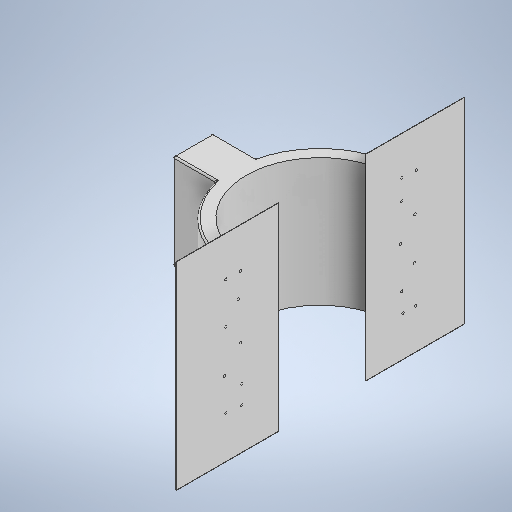
# Autodesk Inventor part: moror-mount1
Saved by Autodesk Inventor 2025.2 (Build 292293000, 293)
## iProperties
Created: 2025-02-07
Part Number: moror-mount1
Material: 一般
Document SubType Name: Modeling
Designer: mahhy
Density: 1 g/cm^3
Appearance: 既定
Author: mahhy
## iProperties of the stored document moror-mount1_3D プリント.ipt
Created: 2025-02-16
Part Number: moror-mount1_3D プリント
Material: 一般
Document SubType Name: Modeling
Designer: mahhy
Density: 1 g/cm^3
Appearance: 既定
Author: mahhy
Autodesk Inventor part; units mm, degrees
ref_plane "YZ Plane" through (0, 0, 0) normal (1, 0, 0) x (0, 1, 0)
ref_plane "XZ Plane" through (0, 0, 0) normal (0, 1, 0) x (-1, 0, 0)
ref_plane "XY Plane" through (0, 0, 0) normal (0, 0, 1) x (1, 0, 0)
sketch "スケッチ1" plane through (0, 0, 0) normal (0, 1, 0) x (-1, 0, 0)
  line L0 (0, 0) -> (60, 0)
  line L1 (60, 0) -> (60, -120)
  line L2 (60, -120) -> (0, -120)
  line L3 (0, -120) -> (0, 0)
  circle A0 centre (0, -60) radius 46
  circle A1 centre (0, -60) radius 54
  line L4 (0, -14) -> (7, -14)
  line L5 (7, -14) -> (7, 4)
  line L6 (7, 4) -> (0, 4)
  line L7 (0, 4) -> (0, -14)
  line L8 (0, -106) -> (7, -106)
  line L9 (7, -106) -> (7, -124)
  line L10 (7, -124) -> (0, -124)
  line L11 (0, -124) -> (0, -106)
  line L12 (54, -47.5) -> (46, -47.5)
  line L13 (46, -47.5) -> (46, -72.5)
  line L14 (46, -72.5) -> (54, -72.5)
  line L15 (54, -72.5) -> (54, -47.5)
  point P0 (46, -60)
  point P1 (52.5333, -47.5)
  point P2 (7, -6.4556)
  point P3 (0, -2)
  point P4 (0, -118)
  point P5 (7, -113.5444)
  point P6 (52.5333, -72.5)
  point P7 (7, 0)
  point P8 (7, -120)
  point P9 (54, -60)
  point P10 (0, -114)
  point P11 (0, -6)
  dimension "d2" = 60
  dimension "d3" = 120
  dimension "d4" = 92
  dimension "d5" = 108
  dimension "d6" = 7
  dimension "d7" = 18
  dimension "d8" = 7
  dimension "d9" = 18
  dimension "d10" = 8
  dimension "d11" = 25
  dimension "d38" = 0
  constraints: 32 end point, 8 parallel, 4 horizontal, 4 perpendicular, 3 point on circle, 2 centre point, 2 midpoint, 2 point on line, 1 coincident
  measures "d2" distance of L1.end L2.end
  measures "d3" distance of L0.end L1.end
  measures "d4" diameter of A0
  measures "d5" diameter of A1
  measures "d6" distance of L6.end L5.end
  measures "d7" distance of L5.end L4.end
  measures "d8" distance of L9.end L10.end
  measures "d9" distance of L8.end L9.end
  measures "d10" distance of L14.end L13.end
  measures "d11" distance of L13.end L12.end
  measures "d38" vertical distance of A0.centre point (46, -60)
extrude "押し出し1" add sketch "スケッチ1" along normal blind 80 contours L7 L6 L5 L0 | L0 L5 A1 L3 | A1 L5 L4 L3 | A1 L12 L13 A0 L4 L5 | A1 L9 L2 L3 | L3 L8 L9 A1 | L12 L15 A1 | A1 L14 L13 L12 | A0 L13 L14 A1 L9 L8 | L2 L9 L10 L11 | L15 L14 A1
sketch "スケッチ2" plane through (-54, 0, -72.5) normal (-1, 0, 0) x (0, 0, 1)
  line L0 (25, 0) -> (25, 80) projected
  line L1 (0, 20) -> (25, 20)
  line L2 (25, 20) -> (25, 80)
  line L3 (25, 80) -> (0, 80)
  line L4 (0, 80) -> (0, 20)
  line L5 (0, 0) -> (25, 0) projected
  line L6 (2.2, 30.1) -> (22.8, 30.1)
  line L7 (22.8, 30.1) -> (22.8, 71.1)
  line L8 (22.8, 71.1) -> (2.2, 71.1)
  line L9 (2.2, 71.1) -> (2.2, 30.1)
  line L10 (-33.5, 80) -> (58.5, 80) projected
  point P0 (72.5, 0)
  point P1 (12.5, 40)
  point P2 (12.5, 71.1)
  point P3 (12.5, 80)
  point P4 (12.5, 80)
  point P5 (25, 20)
  point P6 (12.5, 0)
  dimension "d14" = 25
  dimension "d15" = 60
  dimension "d16" = 40
  dimension "d17" = 20.6
  dimension "d18" = 0
  dimension "d19" = 41
  dimension "d20" = 9.9
  constraints: 16 end point, 4 parallel, 3 midpoint, 2 horizontal, 2 perpendicular
  measures "d14" distance of L3.end L0.end
  measures "d15" distance of L0.end L1.end
  measures "d16" distance from line of L5 point (12.5, 40)
  measures "d17" distance of L8.end L7.end
  measures "d18" horizontal distance of point (12.5, 80) point (12.5, 71.1)
  measures "d19" distance between parallel lines of L8 L6
  measures "d20" distance from line of point (12.5, 40) L6
extrude "押し出し2" add sketch "スケッチ2" along normal blind 25.5
sketch "スケッチ3" plane through (-79.5, 0, -72.5) normal (-1, 0, 0) x (0, 0, 1)
  line L0 (2.2, 71.1) -> (22.8, 71.1) projected
  line L1 (22.8, 30.1) -> (2.2, 30.1) projected
  line L2 (7.65, 75.1) -> (17.35, 75.1)
  line L3 (7.65, 26.1) -> (17.35, 26.1)
  point P0 (72.5, 0)
  point P1 (12.5, 75.1)
  point P2 (12.5, 26.1)
  point P3 (12.5, 71.1)
  point P4 (12.5, 30.1)
  dimension "d23" = 9.7
  dimension "d24" = 9.7
  dimension "d25" = 0
  dimension "d26" = 0
  dimension "d27" = 4
  dimension "d28" = 4
  dimension "d29" = 0
  dimension "d30" = 0
  constraints: 4 end point, 4 midpoint
  measures "d23" distance of L2.end L2.start
  measures "d24" distance of L3.end L3.start
  measures "d25" vertical distance of L2.start L2.end
  measures "d26" vertical distance of L3.start L3.end
  measures "d27" distance from line of L0 L2.start
  measures "d28" distance from line of L1 L3.end
  measures "d29" horizontal distance of point (12.5, 71.1) point (12.5, 75.1)
  measures "d30" horizontal distance of point (12.5, 30.1) point (12.5, 26.1)
hole "穴1" at (-79.5, 75.1, -64.85) at (-79.5, 75.1, -55.15) at (-79.5, 26.1, -55.15) at (-79.5, 26.1, -64.85) direction (1, 0, 0) diameter 4 depth 5
sketch "スケッチ5" plane through (-7, 0, -124) normal (-1, 0, 0) x (0, 0, 1)
  line L0 (0, 80) -> (10.4556, 80) projected
  line L1 (18, 0) -> (0, 0) projected
  line L2 (128, 80) -> (110, 80) projected
  line L3 (117.5444, 0) -> (128, 0) projected
  line L4 (117.5444, 80) -> (128, 80) projected
  line L5 (0, 0) -> (10.4556, 0) projected
  point P0 (5.2278, 80)
  point P1 (5.2278, 70)
  point P2 (122.7722, 70)
  point P3 (122.7722, 10)
  point P4 (5.2278, 80)
  point P5 (122.7722, 0)
  point P6 (122.7722, 80)
  point P7 (5.2278, 80)
  point P8 (122.7722, 80)
  point P9 (122.7722, 0)
  point P10 (5.2278, 10)
  point P11 (5.2278, 0)
  dimension "d56" = 10
  dimension "d58" = 10
  dimension "d59" = 10
  dimension "d67" = 0
  dimension "d68" = 0
  dimension "d69" = 0
  dimension "d70" = 10
  constraints: 8 midpoint
  measures "d56" distance of point (5.228, 80) point (5.228, 70)
  measures "d58" distance of point (122.772, 0) point (122.772, 10)
  measures "d59" distance of point (122.772, 70) point (122.772, 80)
  measures "d67" horizontal distance of point (5.228, 70) point (5.228, 80)
  measures "d68" horizontal distance of point (122.772, 70) point (122.772, 80)
  measures "d69" horizontal distance of point (122.772, 0) point (122.772, 10)
  measures "d70" distance of point (5.228, 0) point (5.228, 10)
hole "穴3" at (-7, 70, -118.7722) at (-7, 10, -1.2278) at (-7, 70, -1.2278) at (-7, 10, -118.7722) direction (1, 0, 0) diameter 4.2 end through all
fillet "フィレット1" radius 1 14 edges at (-3.5, 80, -124) (-7, 80, -118.7722) (-7, 40, -124) (-7, 0, -118.7722) (-3.5, 0, -124) (-36.1554, 80, -100.1097) (-36.1554, 0, -100.1097) (-36.1554, 80, -19.8903) (-7, 80, -1.2278) (-3.5, 80, 4) (-7, 40, 4) (-36.1554, 0, -19.8903) (-7, 0, -1.2278) (-3.5, 0, 4)
fillet "フィレット2" radius 2 1 edges at (-54, 0, -60)
fillet "フィレット4" radius 1 10 edges at (-79.5, 50, -47.5) (-79.5, 80, -60) (-79.5, 50, -72.5) (-79.5, 20, -60) (-66.75, 20, -47.5) (-52.0191, 80, -47.5) (-66.0167, 80, -47.5) (-66.75, 20, -72.5) (-52.0191, 80, -72.5) (-66.0167, 80, -72.5)
fillet "フィレット5" radius 1 12 edges at (-52.2762, 79.7376, -72.1753) (-52.2296, 0.2903, -72.5) (-52.5333, 40, -72.5) (-6.669, 79.7433, -113.253) (-6.669, 0.2567, -113.253) (-7, 40, -113.5444) (-52.2762, 79.7375, -47.8247) (-52.2296, 0.2903, -47.5) (-52.5333, 40, -47.5) (-6.669, 79.7433, -6.747) (-6.669, 0.2567, -6.747) (-7, 40, -6.4556)
sketch "スケッチ6" plane through (-54, 30.1, -49.7) normal (-1, 0, 0) x (0, 0, 1)
  line L0 (-20.6, 41) -> (-20.6, 0) projected
  line L1 (0, 0) -> (0, 41) projected
  line L2 (-20.6, 41) -> (0, 41)
  line L3 (0, 41) -> (0, 0)
  line L4 (0, 0) -> (-20.6, 0)
  line L5 (-20.6, 0) -> (-20.6, 41)
  point P0 (49.7, -30.1)
  point P1 (0, 41)
  point P2 (-20.6, 0)
  constraints: 8 end point, 2 parallel, 1 horizontal, 1 perpendicular
extrude "押し出し3" cut sketch "スケッチ6" against normal blind 2
sketch "スケッチ7" plane through (0, 0, -14) normal (1, 0, 0) x (0, 0, -1)
  circle A0 centre (-4.4271, 76.7147) radius 0.75
  circle A1 centre (-13.6406, 76.7147) radius 0.75
  circle A2 centre (-5.994, 62.0652) radius 0.75
  circle A3 centre (-13.6406, 51.0898) radius 0.75
  circle A4 centre (-4.4271, 37.8359) radius 0.75
  circle A5 centre (-14.3906, 24.7807) radius 0.75
  circle A6 centre (-3.6771, 3.5122) radius 0.75
  circle A7 centre (-13.6406, 4.2622) radius 0.75
  circle A8 centre (-3.6771, 15.1477) radius 0.75
  circle A9 centre (105.2497, 3.0105) radius 0.75
  circle A10 centre (97.2757, 3.0105) radius 0.75
  circle A11 centre (96.5257, 15.1477) radius 0.75
  circle A12 centre (104.4083, 26.7742) radius 0.75
  circle A13 centre (95.7757, 41.3033) radius 0.75
  circle A14 centre (104.7657, 52.8326) radius 0.75
  circle A15 centre (96.5257, 76.7147) radius 0.75
  circle A16 centre (105.5157, 76.4199) radius 0.75
  circle A17 centre (96.5257, 64.0472) radius 0.75
  point P0 (-14, 0)
  dimension "d78" = 1.5
  dimension "d79" = 1.5
  dimension "d80" = 1.5
  dimension "d81" = 1.5
  dimension "d82" = 1.5
  dimension "d83" = 1.5
  dimension "d84" = 1.5
  dimension "d85" = 1.5
  dimension "d86" = 1.5
  dimension "d87" = 1.5
  dimension "d88" = 1.5
  dimension "d89" = 1.5
  dimension "d90" = 1.5
  dimension "d91" = 1.5
  dimension "d92" = 1.5
  dimension "d93" = 1.5
  dimension "d94" = 1.5
  dimension "d95" = 1.5
  constraints: 18 centre point
  measures "d78" diameter of A0
  measures "d79" diameter of A1
  measures "d80" diameter of A2
  measures "d81" diameter of A3
  measures "d82" diameter of A4
  measures "d83" diameter of A5
  measures "d84" diameter of A6
  measures "d85" diameter of A7
  measures "d86" diameter of A8
  measures "d87" diameter of A9
  measures "d88" diameter of A10
  measures "d89" diameter of A11
  measures "d90" diameter of A12
  measures "d91" diameter of A13
  measures "d92" diameter of A14
  measures "d93" diameter of A15
  measures "d94" diameter of A16
  measures "d95" diameter of A17
extrude "押し出し4" add sketch "スケッチ7" along normal blind 0.8
sketch "スケッチ8" plane through (0.8, 62.0652, -8.006) normal (1, 0, 0) x (0, 0, -1)
  line L0 (-38.8707, 39.8297) -> (25.4196, 39.8297)
  line L1 (25.4196, 39.8297) -> (25.4196, -84.0964)
  line L2 (25.4196, -84.0964) -> (-38.8707, -84.0964)
  line L3 (-38.8707, -84.0964) -> (-38.8707, 39.8297)
  line L4 (79.8946, 38.8737) -> (141.4516, 38.8737)
  line L5 (141.4516, 38.8737) -> (141.4516, -84.0794)
  line L6 (141.4516, -84.0794) -> (79.8946, -84.0794)
  line L7 (79.8946, -84.0794) -> (79.8946, 38.8737)
  point P0 (-8.006, -62.0652)
  constraints: 16 end point, 4 parallel, 2 horizontal, 2 perpendicular
extrude "押し出し5" add sketch "スケッチ8" along normal blind 0.2
